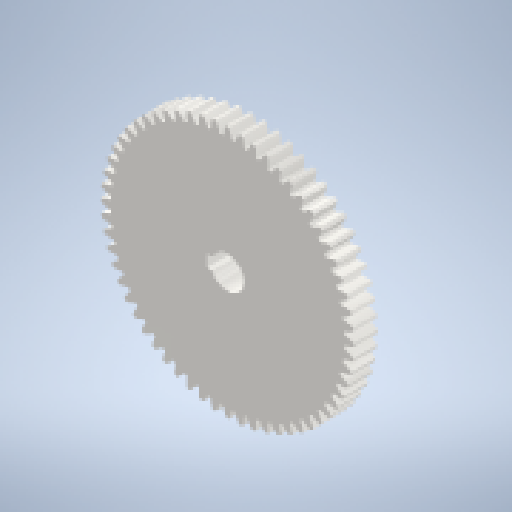
# Autodesk Inventor part: 平歯車1
Saved by Autodesk Inventor 2024 (Build 280153000, 153)
## iProperties
Created: 2023-05-30
Part Number: 平歯車1
Material: Steel
Document SubType Name: Modeling
Designer: yuta2
Categories: <?xml version="1.0" encoding="UTF-16"?> <MemberInstance><Categories><FamilyTemplate><FamilyTemplateParameter ValueType="xs:double" Id="1" ObjectReferenceKey="da_z" ObjectType="kUserParameterObject"/><FamilyTemplateParameter ValueType="xs:double" Id="2" ObjectReferenceKey="da_b" ObjectType="kUserParameterObject"/><FamilyTemplateParameter ValueType="xs:double" Id="3" ObjectReferenceKey="da_beta" ObjectType="kUserParameterObject"/><FamilyTemplateParameter ValueType="xs:double" Id="4" ObjectReferenceKey="da_da" ObjectType="kUserParameterObject"/><FamilyTemplateParameter ValueType="xs:double" Id="5" ObjectReferenceKey="da_aw" ObjectType="kUserParameterObject"/><FamilyTemplateParameter ValueType="xs:string" Id="6" ObjectReferenceKey="EAIAABAAAACIAQAAAAAAAIAAAAAAAAAA" ObjectType="83910656" SubObjectId="SurfaceGeometry"/></FamilyTemplate><ParamToTemplateMap><ParamToTemplate CategoryParameter="//CategoryParameter[@InternalName='046C89C9-8512-4d59-83FE-43B91F4F132A']" TemplateParameter="1"/><ParamToTemplate CategoryParameter="//CategoryParameter[@InternalName='2552DF32-E462-4b46-AEBF-C6C7768E72AC']" TemplateParameter="2"/><ParamToTemplate CategoryParameter="//CategoryParameter[@InternalName='C9EE641D-15FC-4fae-A226-E94C4372FDD7']" TemplateParameter="3"/><ParamToTemplate><ParamToTemplate CategoryParameter="//CategoryParameter[@InternalName='00B6519A-459B-49c7-AD84-2E56D39A5744']" ConstantValue="0.000000"/></ParamToTemplate><ParamToTemplate><ParamToTemplate CategoryParameter="//CategoryParameter[@InternalName='04B31F0E-C7A6-4894-AA32-9629BEFACF47']" ConstantValue="1.000000"/></ParamToTemplate><ParamToTemplate><ParamToTemplate CategoryParameter="//CategoryParameter[@InternalName='43CBEC2E-7847-49e7-A936-2F7889FCB2D9']" ConstantValue="0.250000"/></ParamToTemplate><ParamToTemplate><ParamToTemplate CategoryParameter="//CategoryParameter[@InternalName='B1EFC894-105D-4ebd-86BF-FA20ED196853']" ConstantValue="0.350000"/></ParamToTemplate><ParamToTemplate><ParamToTemplate CategoryParameter="//CategoryParameter[@InternalName='51175063-3D10-4879-93E8-6246FE8B403D']" ConstantValue="2060000000.000000"/></ParamToTemplate><ParamToTemplate><ParamToTemplate CategoryParameter="//CategoryParameter[@InternalName='A3A52E27-4454-46a9-B0BD-C932399B70AF']" ConstantValue="0.300000"/></ParamToTemplate><ParamToTemplate><ParamToTemplate CategoryParameter="//CategoryParameter[@InternalName='91B76062-C214-41d9-B1B9-14D2AB99603D']" ConstantValue="0.100000"/></ParamToTemplate><ParamToTemplate><ParamToTemplate CategoryParameter="//CategoryParameter[@InternalName='374E806E-8B8A-4dda-A9AA-1039D6500AD2']" ConstantValue="10.000000"/></ParamToTemplate><ParamToTemplate><ParamToTemplate CategoryParameter="//CategoryParameter[@InternalName='2D373A89-B862-43d6-8D0B-0CBF12AB9F6C']" ConstantValue="0.349066"/></ParamToTemplate><ParamToTemplate CategoryParameter="//CategoryParameter[@InternalName='37777632-D6A2-4fac-9D53-DB8ACD95C989']" TemplateParameter="4"/><ParamToTemplate CategoryParameter="//CategoryParameter[@InternalName='FD1017F1-B727-4f7e-9707-0F86F1FF9423']" TemplateParameter="5"/><ParamToTemplate><ParamToTemplate CategoryParameter="//CategoryParameter[@InternalName='9E1B4470-B2D3-4ff1-B813-535BB4CDF51A']" ConstantValue="3520000.000000"/></ParamToTemplate><ParamToTemplate><ParamToTemplate CategoryParameter="//CategoryParameter[@InternalName='F8452263-BFF6-458c-9FB1-07C4B99E95CD']" ConstantValue="11400000.000000"/></ParamToTemplate><ParamToTemplate><ParamToTemplate CategoryParameter="//CategoryParameter[@InternalName='3E3BB259-FD49-497f-8171-6EBC954A3479']" ConstantValue="2.000000"/></ParamToTemplate><ParamToTemplate CategoryParameter="//CategoryParameter[@InternalName='27C3BAF2-7550-4e4b-AE2C-0DB134B7D9B7']" TemplateParameter="6"/></ParamToTemplateMap><Category DisplayName="Gear" InternalName="DC85795E-93AB-48d5-8EEE-5A27447B64BD" Mnemonic="Gear"><CategoryParameter DisplayName="z" InternalName="046C89C9-8512-4d59-83FE-43B91F4F132A" Mnemonic="z"/><CategoryParameter DisplayName="b" InternalName="2552DF32-E462-4b46-AEBF-C6C7768E72AC" Mnemonic="b"/><CategoryParameter DisplayName="||b|" InternalName="C9EE641D-15FC-4fae-A226-E94C4372FDD7" Mnemonic="beta"/><CategoryParameter DisplayName="x" InternalName="00B6519A-459B-49c7-AD84-2E56D39A5744" Mnemonic="x"/><CategoryParameter DisplayName="a*" InternalName="04B31F0E-C7A6-4894-AA32-9629BEFACF47" Mnemonic="a"/><CategoryParameter DisplayName="c*" InternalName="43CBEC2E-7847-49e7-A936-2F7889FCB2D9" Mnemonic="c"/><CategoryParameter DisplayName="r|.f|*" InternalName="B1EFC894-105D-4ebd-86BF-FA20ED196853" Mnemonic="rf"/><CategoryParameter DisplayName="E" InternalName="51175063-3D10-4879-93E8-6246FE8B403D" Mnemonic="E"/><CategoryParameter DisplayName="||m|" InternalName="A3A52E27-4454-46a9-B0BD-C932399B70AF" Mnemonic="mi"/><Category DisplayName="SpurGear" InternalName="26C5A22E-A91E-4dfd-A3B3-23CCAFAE1764" Mnemonic="SpurGear"><CategoryParameter DisplayName="m" InternalName="91B76062-C214-41d9-B1B9-14D2AB99603D" Mnemonic="m"/><CategoryParameter DisplayName="P" InternalName="374E806E-8B8A-4dda-A9AA-1039D6500AD2" Mnemonic="PP"/><CategoryParameter DisplayName="||a|" InternalName="2D373A89-B862-43d6-8D0B-0CBF12AB9F6C" Mnemonic="alpha"/><CategoryParameter DisplayName="d|.a|" InternalName="37777632-D6A2-4fac-9D53-DB8ACD95C989" Mnemonic="da"/><CategoryParameter DisplayName="a|.w|" InternalName="FD1017F1-B727-4f7e-9707-0F86F1FF9423" Mnemonic="aw"/><CategoryParameter DisplayName="||s||.Flim|" InternalName="9E1B4470-B2D3-4ff1-B813-535BB4CDF51A" Mnemonic="sFlim"/><CategoryParameter DisplayName="||s||.Hlim|" InternalName="F8452263-BFF6-458c-9FB1-07C4B99E95CD" Mnemonic="sHlim"/><CategoryParameter DisplayName="タイプ" InternalName="3E3BB259-FD49-497f-8171-6EBC954A3479" Mnemonic="type"/><CategoryParameter DisplayName="PitchDiameter" InternalName="27C3BAF2-7550-4e4b-AE2C-0DB134B7D9B7" Mnemonic="IDS_PITCHDIAM"/></Category></Category></Categories></MemberInstance>
Density: 1 g/cm^3
Appearance: Steel
CustomPartVersion: 1
Author: yuta2
Autodesk Inventor part; units mm, degrees
sketch "Sketch1" plane through (0, 0, 0) normal (0, 0, 1) x (1, 0, 0)
  circle A0 centre (0, 0) radius 31
  dimension "d0" = 62
  constraints: 1 centre point
  measures "d0" diameter of A0
extrude "Extrusion1" add sketch "Sketch1" along normal blind 6
ref_plane "Work Plane2" through (0, 0, 3) normal (0, 0, 1) x (1, 0, 0)
sketch "Sketch2" plane through (0, 0, 0) normal (0, 0, -1) x (-1, 0, 0)
  circle A0 centre (0, 0) radius 31 projected
  circle A1 centre (0, 0) radius 30
  dimension "d3" = 60
  constraints: 1 centre point, 1 coincident
  measures "d3" diameter of A1
surface extrude "ピッチ円直径" sketch "Sketch2" against normal through all shown no curves A1
ref_plane "Work Plane8" through (0, 0, 0) normal (0.9986295, 0.052336, 0) x (0, 0, 1)
ref_plane "Work Plane9" through (0, 0, 0) normal (1, 0, 0) x (0, 1, 0)
spur gear teeth "平歯車" teeth 60 pitch diameter 60 tip diameter 62 root diameter 57.5 face width 6 start plane through (0, 0, 0) normal (0, 0, -1) x (-1, 0, 0)
sketch "スケッチ3" plane through (0, 0, 0) normal (0, 0, -1) x (-1, 0, 0)
  point P0 (0, 0)
  point P1 (0, 0)
  constraints: 1 coincident
hole "穴1" at (0, 0, 0) direction (0, 0, 1) diameter 8 end through all
sketch "スケッチ4" plane through (0, 0, 0) normal (0, 0, -1) x (-1, 0, 0)
  circle A0 centre (0, 0) radius 4 projected
  arc A1 (4.1254, 28.4525) -> (3.6437, 30.7851) centre (-8.4184, 27.0779) ccw projected
  arc A2 (3.6437, 30.7851) -> (2.8366, 30.87) centre (0, 0) ccw projected
  arc A3 (2.8366, 30.87) -> (1.8803, 28.6884) centre (13.8643, 24.7359) ccw projected
  arc A4 (1.8803, 28.6884) -> (1.1287, 28.7278) centre (0, 0) ccw projected
  arc A5 (1.1287, 28.7278) -> (0.4058, 30.9973) centre (-11.2027, 26.0496) ccw projected
  arc A6 (0.4058, 30.9973) -> (-0.4058, 30.9973) centre (0, 0) ccw projected
  arc A7 (-0.4058, 30.9973) -> (-1.1287, 28.7278) centre (11.2027, 26.0496) ccw projected
  arc A8 (-1.1287, 28.7278) -> (-1.8803, 28.6884) centre (0, 0) ccw projected
  arc A9 (-1.8803, 28.6884) -> (-2.8366, 30.87) centre (-13.8643, 24.7359) ccw projected
  arc A10 (-2.8366, 30.87) -> (-3.6437, 30.7851) centre (0, 0) ccw projected
  arc A11 (-3.6437, 30.7851) -> (-4.1254, 28.4525) centre (8.4184, 27.0779) ccw projected
  arc A12 (-4.1254, 28.4525) -> (-4.8688, 28.3347) centre (0, 0) ccw projected
  arc A13 (-4.8688, 28.3347) -> (-6.0478, 30.4043) centre (-16.3739, 23.1512) ccw projected
  arc A14 (-6.0478, 30.4043) -> (-6.8416, 30.2356) centre (0, 0) ccw projected
  arc A15 (-6.8416, 30.2356) -> (-7.0769, 27.8654) centre (5.5419, 27.8095) ccw projected
  arc A16 (-7.0769, 27.8654) -> (-7.8039, 27.6706) centre (0, 0) ccw projected
  arc A17 (-7.8039, 27.6706) -> (-9.1928, 29.6056) centre (-18.7042, 21.3128) ccw projected
  arc A18 (-9.1928, 29.6056) -> (-9.9646, 29.3548) centre (0, 0) ccw projected
  arc A19 (-9.9646, 29.3548) -> (-9.9509, 26.973) centre (2.6046, 28.2365) ccw projected
  arc A20 (-9.9509, 26.973) -> (-10.6535, 26.7033) centre (0, 0) ccw projected
  arc A21 (-10.6535, 26.7033) -> (-12.2371, 28.4825) centre (-20.8295, 19.241) ccw projected
  arc A22 (-12.2371, 28.4825) -> (-12.9785, 28.1524) centre (0, 0) ccw projected
  arc A23 (-12.9785, 28.1524) -> (-12.7158, 25.7851) centre (-0.3611, 28.3541) ccw projected
  arc A24 (-12.7158, 25.7851) -> (-13.3864, 25.4434) centre (0, 0) ccw projected
  arc A25 (-13.3864, 25.4434) -> (-15.1473, 27.0474) centre (-22.7266, 16.9583) ccw projected
  arc A26 (-15.1473, 27.0474) -> (-15.8501, 26.6416) centre (0, 0) ccw projected
  arc A27 (-15.8501, 26.6416) -> (-15.3414, 24.3147) centre (-3.323, 28.161) ccw projected
  arc A28 (-15.3414, 24.3147) -> (-15.9726, 23.9048) centre (0, 0) ccw projected
  arc A29 (-15.9726, 23.9048) -> (-17.8915, 25.3159) centre (-24.3748, 14.4898) ccw projected
  arc A30 (-17.8915, 25.3159) -> (-18.5481, 24.8389) centre (0, 0) ccw projected
  arc A31 (-18.5481, 24.8389) -> (-17.799, 22.5779) centre (-6.2484, 27.6594) ccw projected
  arc A32 (-17.799, 22.5779) -> (-18.3839, 22.1042) centre (0, 0) ccw projected
  arc A33 (-18.3839, 22.1042) -> (-20.4397, 23.307) centre (-25.7558, 11.8626) ccw projected
  arc A34 (-20.4397, 23.307) -> (-21.0428, 22.764) centre (0, 0) ccw projected
  arc A35 (-21.0428, 22.764) -> (-20.0615, 20.5937) centre (-9.1054, 26.8547) ccw projected
  arc A36 (-20.0615, 20.5937) -> (-20.5937, 20.0615) centre (0, 0) ccw projected
  arc A37 (-20.5937, 20.0615) -> (-22.764, 21.0428) centre (-26.8547, 9.1054) ccw projected
  arc A38 (-22.764, 21.0428) -> (-23.307, 20.4397) centre (0, 0) ccw projected
  arc A39 (-23.307, 20.4397) -> (-22.1042, 18.3839) centre (-11.8626, 25.7558) ccw projected
  arc A40 (-22.1042, 18.3839) -> (-22.5779, 17.799) centre (0, 0) ccw projected
  arc A41 (-22.5779, 17.799) -> (-24.8389, 18.5481) centre (-27.6594, 6.2484) ccw projected
  arc A42 (-24.8389, 18.5481) -> (-25.3159, 17.8915) centre (0, 0) ccw projected
  arc A43 (-25.3159, 17.8915) -> (-23.9048, 15.9726) centre (-14.4898, 24.3748) ccw projected
  arc A44 (-23.9048, 15.9726) -> (-24.3147, 15.3414) centre (0, 0) ccw projected
  arc A45 (-24.3147, 15.3414) -> (-26.6416, 15.8501) centre (-28.161, 3.323) ccw projected
  arc A46 (-26.6416, 15.8501) -> (-27.0474, 15.1473) centre (0, 0) ccw projected
  arc A47 (-27.0474, 15.1473) -> (-25.4434, 13.3864) centre (-16.9583, 22.7266) ccw projected
  arc A48 (-25.4434, 13.3864) -> (-25.7851, 12.7158) centre (0, 0) ccw projected
  arc A49 (-25.7851, 12.7158) -> (-28.1524, 12.9785) centre (-28.3541, 0.3611) ccw projected
  arc A50 (-28.1524, 12.9785) -> (-28.4825, 12.2371) centre (0, 0) ccw projected
  arc A51 (-28.4825, 12.2371) -> (-26.7033, 10.6535) centre (-19.241, 20.8295) ccw projected
  arc A52 (-26.7033, 10.6535) -> (-26.973, 9.9509) centre (0, 0) ccw projected
  arc A53 (-26.973, 9.9509) -> (-29.3548, 9.9646) centre (-28.2365, -2.6046) ccw projected
  arc A54 (-29.3548, 9.9646) -> (-29.6056, 9.1928) centre (0, 0) ccw projected
  arc A55 (-29.6056, 9.1928) -> (-27.6706, 7.8039) centre (-21.3128, 18.7042) ccw projected
  arc A56 (-27.6706, 7.8039) -> (-27.8654, 7.0769) centre (0, 0) ccw projected
  arc A57 (-27.8654, 7.0769) -> (-30.2356, 6.8416) centre (-27.8095, -5.5419) ccw projected
  arc A58 (-30.2356, 6.8416) -> (-30.4043, 6.0478) centre (0, 0) ccw projected
  arc A59 (-30.4043, 6.0478) -> (-28.3347, 4.8688) centre (-23.1512, 16.3739) ccw projected
  arc A60 (-28.3347, 4.8688) -> (-28.4525, 4.1254) centre (0, 0) ccw projected
  arc A61 (-28.4525, 4.1254) -> (-30.7851, 3.6437) centre (-27.0779, -8.4184) ccw projected
  arc A62 (-30.7851, 3.6437) -> (-30.87, 2.8366) centre (0, 0) ccw projected
  arc A63 (-30.87, 2.8366) -> (-28.6884, 1.8803) centre (-24.7359, 13.8643) ccw projected
  arc A64 (-28.6884, 1.8803) -> (-28.7278, 1.1287) centre (0, 0) ccw projected
  arc A65 (-28.7278, 1.1287) -> (-30.9973, 0.4058) centre (-26.0496, -11.2027) ccw projected
  arc A66 (-30.9973, 0.4058) -> (-30.9973, -0.4058) centre (0, 0) ccw projected
  arc A67 (-30.9973, -0.4058) -> (-28.7278, -1.1287) centre (-26.0496, 11.2027) ccw projected
  arc A68 (-28.7278, -1.1287) -> (-28.6884, -1.8803) centre (0, 0) ccw projected
  arc A69 (-28.6884, -1.8803) -> (-30.87, -2.8366) centre (-24.7359, -13.8643) ccw projected
  arc A70 (-30.87, -2.8366) -> (-30.7851, -3.6437) centre (0, 0) ccw projected
  arc A71 (-30.7851, -3.6437) -> (-28.4525, -4.1254) centre (-27.0779, 8.4184) ccw projected
  arc A72 (-28.4525, -4.1254) -> (-28.3347, -4.8688) centre (0, 0) ccw projected
  arc A73 (-28.3347, -4.8688) -> (-30.4043, -6.0478) centre (-23.1512, -16.3739) ccw projected
  arc A74 (-30.4043, -6.0478) -> (-30.2356, -6.8416) centre (0, 0) ccw projected
  arc A75 (-30.2356, -6.8416) -> (-27.8654, -7.0769) centre (-27.8095, 5.5419) ccw projected
  arc A76 (-27.8654, -7.0769) -> (-27.6706, -7.8039) centre (0, 0) ccw projected
  arc A77 (-27.6706, -7.8039) -> (-29.6056, -9.1928) centre (-21.3128, -18.7042) ccw projected
  arc A78 (-29.6056, -9.1928) -> (-29.3548, -9.9646) centre (0, 0) ccw projected
  arc A79 (-29.3548, -9.9646) -> (-26.973, -9.9509) centre (-28.2365, 2.6046) ccw projected
  arc A80 (-26.973, -9.9509) -> (-26.7033, -10.6535) centre (0, 0) ccw projected
  arc A81 (-26.7033, -10.6535) -> (-28.4825, -12.2371) centre (-19.241, -20.8295) ccw projected
  arc A82 (-28.4825, -12.2371) -> (-28.1524, -12.9785) centre (0, 0) ccw projected
  arc A83 (-28.1524, -12.9785) -> (-25.7851, -12.7158) centre (-28.3541, -0.3611) ccw projected
  arc A84 (-25.7851, -12.7158) -> (-25.4434, -13.3864) centre (0, 0) ccw projected
  arc A85 (-25.4434, -13.3864) -> (-27.0474, -15.1473) centre (-16.9583, -22.7266) ccw projected
  arc A86 (-27.0474, -15.1473) -> (-26.6416, -15.8501) centre (0, 0) ccw projected
  arc A87 (-26.6416, -15.8501) -> (-24.3147, -15.3414) centre (-28.161, -3.323) ccw projected
  arc A88 (-24.3147, -15.3414) -> (-23.9048, -15.9726) centre (0, 0) ccw projected
  arc A89 (-23.9048, -15.9726) -> (-25.3159, -17.8915) centre (-14.4898, -24.3748) ccw projected
  arc A90 (-25.3159, -17.8915) -> (-24.8389, -18.5481) centre (0, 0) ccw projected
  arc A91 (-24.8389, -18.5481) -> (-22.5779, -17.799) centre (-27.6594, -6.2484) ccw projected
  arc A92 (-22.5779, -17.799) -> (-22.1042, -18.3839) centre (0, 0) ccw projected
  arc A93 (-22.1042, -18.3839) -> (-23.307, -20.4397) centre (-11.8626, -25.7558) ccw projected
  arc A94 (-23.307, -20.4397) -> (-22.764, -21.0428) centre (0, 0) ccw projected
  arc A95 (-22.764, -21.0428) -> (-20.5937, -20.0615) centre (-26.8547, -9.1054) ccw projected
  arc A96 (-20.5937, -20.0615) -> (-20.0615, -20.5937) centre (0, 0) ccw projected
  arc A97 (-20.0615, -20.5937) -> (-21.0428, -22.764) centre (-9.1054, -26.8547) ccw projected
  arc A98 (-21.0428, -22.764) -> (-20.4397, -23.307) centre (0, 0) ccw projected
  arc A99 (-20.4397, -23.307) -> (-18.3839, -22.1042) centre (-25.7558, -11.8626) ccw projected
  arc A100 (-18.3839, -22.1042) -> (-17.799, -22.5779) centre (0, 0) ccw projected
  arc A101 (-17.799, -22.5779) -> (-18.5481, -24.8389) centre (-6.2484, -27.6594) ccw projected
  arc A102 (-18.5481, -24.8389) -> (-17.8915, -25.3159) centre (0, 0) ccw projected
  arc A103 (-17.8915, -25.3159) -> (-15.9726, -23.9048) centre (-24.3748, -14.4898) ccw projected
  arc A104 (-15.9726, -23.9048) -> (-15.3414, -24.3147) centre (0, 0) ccw projected
  arc A105 (-15.3414, -24.3147) -> (-15.8501, -26.6416) centre (-3.323, -28.161) ccw projected
  arc A106 (-15.8501, -26.6416) -> (-15.1473, -27.0474) centre (0, 0) ccw projected
  arc A107 (-15.1473, -27.0474) -> (-13.3864, -25.4434) centre (-22.7266, -16.9583) ccw projected
  arc A108 (-13.3864, -25.4434) -> (-12.7158, -25.7851) centre (0, 0) ccw projected
  arc A109 (-12.7158, -25.7851) -> (-12.9785, -28.1524) centre (-0.3611, -28.3541) ccw projected
  arc A110 (-12.9785, -28.1524) -> (-12.2371, -28.4825) centre (0, 0) ccw projected
  arc A111 (-12.2371, -28.4825) -> (-10.6535, -26.7033) centre (-20.8295, -19.241) ccw projected
  arc A112 (-10.6535, -26.7033) -> (-9.9509, -26.973) centre (0, 0) ccw projected
  arc A113 (-9.9509, -26.973) -> (-9.9646, -29.3548) centre (2.6046, -28.2365) ccw projected
  arc A114 (-9.9646, -29.3548) -> (-9.1928, -29.6056) centre (0, 0) ccw projected
  arc A115 (-9.1928, -29.6056) -> (-7.8039, -27.6706) centre (-18.7042, -21.3128) ccw projected
  arc A116 (-7.8039, -27.6706) -> (-7.0769, -27.8654) centre (0, 0) ccw projected
  arc A117 (-7.0769, -27.8654) -> (-6.8416, -30.2356) centre (5.5419, -27.8095) ccw projected
  arc A118 (-6.8416, -30.2356) -> (-6.0478, -30.4043) centre (0, 0) ccw projected
  arc A119 (-6.0478, -30.4043) -> (-4.8688, -28.3347) centre (-16.3739, -23.1512) ccw projected
  arc A120 (-4.8688, -28.3347) -> (-4.1254, -28.4525) centre (0, 0) ccw projected
  arc A121 (-4.1254, -28.4525) -> (-3.6437, -30.7851) centre (8.4184, -27.0779) ccw projected
  arc A122 (-3.6437, -30.7851) -> (-2.8366, -30.87) centre (0, 0) ccw projected
  arc A123 (-2.8366, -30.87) -> (-1.8803, -28.6884) centre (-13.8643, -24.7359) ccw projected
  arc A124 (-1.8803, -28.6884) -> (-1.1287, -28.7278) centre (0, 0) ccw projected
  arc A125 (-1.1287, -28.7278) -> (-0.4058, -30.9973) centre (11.2027, -26.0496) ccw projected
  arc A126 (-0.4058, -30.9973) -> (0.4058, -30.9973) centre (0, 0) ccw projected
  arc A127 (0.4058, -30.9973) -> (1.1287, -28.7278) centre (-11.2027, -26.0496) ccw projected
  arc A128 (1.1287, -28.7278) -> (1.8803, -28.6884) centre (0, 0) ccw projected
  arc A129 (1.8803, -28.6884) -> (2.8366, -30.87) centre (13.8643, -24.7359) ccw projected
  arc A130 (2.8366, -30.87) -> (3.6437, -30.7851) centre (0, 0) ccw projected
  arc A131 (3.6437, -30.7851) -> (4.1254, -28.4525) centre (-8.4184, -27.0779) ccw projected
  arc A132 (4.1254, -28.4525) -> (4.8688, -28.3347) centre (0, 0) ccw projected
  arc A133 (4.8688, -28.3347) -> (6.0478, -30.4043) centre (16.3739, -23.1512) ccw projected
  arc A134 (6.0478, -30.4043) -> (6.8416, -30.2356) centre (0, 0) ccw projected
  arc A135 (6.8416, -30.2356) -> (7.0769, -27.8654) centre (-5.5419, -27.8095) ccw projected
  arc A136 (7.0769, -27.8654) -> (7.8039, -27.6706) centre (0, 0) ccw projected
  arc A137 (7.8039, -27.6706) -> (9.1928, -29.6056) centre (18.7042, -21.3128) ccw projected
  arc A138 (9.1928, -29.6056) -> (9.9646, -29.3548) centre (0, 0) ccw projected
  arc A139 (9.9646, -29.3548) -> (9.9509, -26.973) centre (-2.6046, -28.2365) ccw projected
  arc A140 (9.9509, -26.973) -> (10.6535, -26.7033) centre (0, 0) ccw projected
  arc A141 (10.6535, -26.7033) -> (12.2371, -28.4825) centre (20.8295, -19.241) ccw projected
  arc A142 (12.2371, -28.4825) -> (12.9785, -28.1524) centre (0, 0) ccw projected
  arc A143 (12.9785, -28.1524) -> (12.7158, -25.7851) centre (0.3611, -28.3541) ccw projected
  arc A144 (12.7158, -25.7851) -> (13.3864, -25.4434) centre (0, 0) ccw projected
  arc A145 (13.3864, -25.4434) -> (15.1473, -27.0474) centre (22.7266, -16.9583) ccw projected
  arc A146 (15.1473, -27.0474) -> (15.8501, -26.6416) centre (0, 0) ccw projected
  arc A147 (15.8501, -26.6416) -> (15.3414, -24.3147) centre (3.323, -28.161) ccw projected
  arc A148 (15.3414, -24.3147) -> (15.9726, -23.9048) centre (0, 0) ccw projected
  arc A149 (15.9726, -23.9048) -> (17.8915, -25.3159) centre (24.3748, -14.4898) ccw projected
  arc A150 (17.8915, -25.3159) -> (18.5481, -24.8389) centre (0, 0) ccw projected
  arc A151 (18.5481, -24.8389) -> (17.799, -22.5779) centre (6.2484, -27.6594) ccw projected
  arc A152 (17.799, -22.5779) -> (18.3839, -22.1042) centre (0, 0) ccw projected
  arc A153 (18.3839, -22.1042) -> (20.4397, -23.307) centre (25.7558, -11.8626) ccw projected
  arc A154 (20.4397, -23.307) -> (21.0428, -22.764) centre (0, 0) ccw projected
  arc A155 (21.0428, -22.764) -> (20.0615, -20.5937) centre (9.1054, -26.8547) ccw projected
  arc A156 (20.0615, -20.5937) -> (20.5937, -20.0615) centre (0, 0) ccw projected
  arc A157 (20.5937, -20.0615) -> (22.764, -21.0428) centre (26.8547, -9.1054) ccw projected
  arc A158 (22.764, -21.0428) -> (23.307, -20.4397) centre (0, 0) ccw projected
  arc A159 (23.307, -20.4397) -> (22.1042, -18.3839) centre (11.8626, -25.7558) ccw projected
  arc A160 (22.1042, -18.3839) -> (22.5779, -17.799) centre (0, 0) ccw projected
  arc A161 (22.5779, -17.799) -> (24.8389, -18.5481) centre (27.6594, -6.2484) ccw projected
  arc A162 (24.8389, -18.5481) -> (25.3159, -17.8915) centre (0, 0) ccw projected
  arc A163 (25.3159, -17.8915) -> (23.9048, -15.9726) centre (14.4898, -24.3748) ccw projected
  arc A164 (23.9048, -15.9726) -> (24.3147, -15.3414) centre (0, 0) ccw projected
  arc A165 (24.3147, -15.3414) -> (26.6416, -15.8501) centre (28.161, -3.323) ccw projected
  arc A166 (26.6416, -15.8501) -> (27.0474, -15.1473) centre (0, 0) ccw projected
  arc A167 (27.0474, -15.1473) -> (25.4434, -13.3864) centre (16.9583, -22.7266) ccw projected
  arc A168 (25.4434, -13.3864) -> (25.7851, -12.7158) centre (0, 0) ccw projected
  arc A169 (25.7851, -12.7158) -> (28.1524, -12.9785) centre (28.3541, -0.3611) ccw projected
  arc A170 (28.1524, -12.9785) -> (28.4825, -12.2371) centre (0, 0) ccw projected
  arc A171 (28.4825, -12.2371) -> (26.7033, -10.6535) centre (19.241, -20.8295) ccw projected
  arc A172 (26.7033, -10.6535) -> (26.973, -9.9509) centre (0, 0) ccw projected
  arc A173 (26.973, -9.9509) -> (29.3548, -9.9646) centre (28.2365, 2.6046) ccw projected
  arc A174 (29.3548, -9.9646) -> (29.6056, -9.1928) centre (0, 0) ccw projected
  arc A175 (29.6056, -9.1928) -> (27.6706, -7.8039) centre (21.3128, -18.7042) ccw projected
  arc A176 (27.6706, -7.8039) -> (27.8654, -7.0769) centre (0, 0) ccw projected
  arc A177 (27.8654, -7.0769) -> (30.2356, -6.8416) centre (27.8095, 5.5419) ccw projected
  arc A178 (30.2356, -6.8416) -> (30.4043, -6.0478) centre (0, 0) ccw projected
  arc A179 (30.4043, -6.0478) -> (28.3347, -4.8688) centre (23.1512, -16.3739) ccw projected
  arc A180 (28.3347, -4.8688) -> (28.4525, -4.1254) centre (0, 0) ccw projected
  arc A181 (28.4525, -4.1254) -> (30.7851, -3.6437) centre (27.0779, 8.4184) ccw projected
  arc A182 (30.7851, -3.6437) -> (30.87, -2.8366) centre (0, 0) ccw projected
  arc A183 (30.87, -2.8366) -> (28.6884, -1.8803) centre (24.7359, -13.8643) ccw projected
  arc A184 (28.6884, -1.8803) -> (28.7278, -1.1287) centre (0, 0) ccw projected
  arc A185 (28.7278, -1.1287) -> (30.9973, -0.4058) centre (26.0496, 11.2027) ccw projected
  arc A186 (30.9973, -0.4058) -> (30.9973, 0.4058) centre (0, 0) ccw projected
  arc A187 (30.9973, 0.4058) -> (28.7278, 1.1287) centre (26.0496, -11.2027) ccw projected
  arc A188 (28.7278, 1.1287) -> (28.6884, 1.8803) centre (0, 0) ccw projected
  arc A189 (28.6884, 1.8803) -> (30.87, 2.8366) centre (24.7359, 13.8643) ccw projected
  arc A190 (30.87, 2.8366) -> (30.7851, 3.6437) centre (0, 0) ccw projected
  arc A191 (30.7851, 3.6437) -> (28.4525, 4.1254) centre (27.0779, -8.4184) ccw projected
  arc A192 (28.4525, 4.1254) -> (28.3347, 4.8688) centre (0, 0) ccw projected
  arc A193 (28.3347, 4.8688) -> (30.4043, 6.0478) centre (23.1512, 16.3739) ccw projected
  arc A194 (30.4043, 6.0478) -> (30.2356, 6.8416) centre (0, 0) ccw projected
  arc A195 (30.2356, 6.8416) -> (27.8654, 7.0769) centre (27.8095, -5.5419) ccw projected
  arc A196 (27.8654, 7.0769) -> (27.6706, 7.8039) centre (0, 0) ccw projected
  arc A197 (27.6706, 7.8039) -> (29.6056, 9.1928) centre (21.3128, 18.7042) ccw projected
  arc A198 (29.6056, 9.1928) -> (29.3548, 9.9646) centre (0, 0) ccw projected
  arc A199 (29.3548, 9.9646) -> (26.973, 9.9509) centre (28.2365, -2.6046) ccw projected
  arc A200 (26.973, 9.9509) -> (26.7033, 10.6535) centre (0, 0) ccw projected
  arc A201 (26.7033, 10.6535) -> (28.4825, 12.2371) centre (19.241, 20.8295) ccw projected
  arc A202 (28.4825, 12.2371) -> (28.1524, 12.9785) centre (0, 0) ccw projected
  arc A203 (28.1524, 12.9785) -> (25.7851, 12.7158) centre (28.3541, 0.3611) ccw projected
  arc A204 (25.7851, 12.7158) -> (25.4434, 13.3864) centre (0, 0) ccw projected
  arc A205 (25.4434, 13.3864) -> (27.0474, 15.1473) centre (16.9583, 22.7266) ccw projected
  arc A206 (27.0474, 15.1473) -> (26.6416, 15.8501) centre (0, 0) ccw projected
  arc A207 (26.6416, 15.8501) -> (24.3147, 15.3414) centre (28.161, 3.323) ccw projected
  arc A208 (24.3147, 15.3414) -> (23.9048, 15.9726) centre (0, 0) ccw projected
  arc A209 (23.9048, 15.9726) -> (25.3159, 17.8915) centre (14.4898, 24.3748) ccw projected
  arc A210 (25.3159, 17.8915) -> (24.8389, 18.5481) centre (0, 0) ccw projected
  arc A211 (24.8389, 18.5481) -> (22.5779, 17.799) centre (27.6594, 6.2484) ccw projected
  arc A212 (22.5779, 17.799) -> (22.1042, 18.3839) centre (0, 0) ccw projected
  arc A213 (22.1042, 18.3839) -> (23.307, 20.4397) centre (11.8626, 25.7558) ccw projected
  arc A214 (23.307, 20.4397) -> (22.764, 21.0428) centre (0, 0) ccw projected
  arc A215 (22.764, 21.0428) -> (20.5937, 20.0615) centre (26.8547, 9.1054) ccw projected
  arc A216 (20.5937, 20.0615) -> (20.0615, 20.5937) centre (0, 0) ccw projected
  arc A217 (20.0615, 20.5937) -> (21.0428, 22.764) centre (9.1054, 26.8547) ccw projected
  arc A218 (21.0428, 22.764) -> (20.4397, 23.307) centre (0, 0) ccw projected
  arc A219 (20.4397, 23.307) -> (18.3839, 22.1042) centre (25.7558, 11.8626) ccw projected
  arc A220 (18.3839, 22.1042) -> (17.799, 22.5779) centre (0, 0) ccw projected
  arc A221 (17.799, 22.5779) -> (18.5481, 24.8389) centre (6.2484, 27.6594) ccw projected
  arc A222 (18.5481, 24.8389) -> (17.8915, 25.3159) centre (0, 0) ccw projected
  arc A223 (17.8915, 25.3159) -> (15.9726, 23.9048) centre (24.3748, 14.4898) ccw projected
  arc A224 (15.9726, 23.9048) -> (15.3414, 24.3147) centre (0, 0) ccw projected
  arc A225 (15.3414, 24.3147) -> (15.8501, 26.6416) centre (3.323, 28.161) ccw projected
  arc A226 (15.8501, 26.6416) -> (15.1473, 27.0474) centre (0, 0) ccw projected
  arc A227 (15.1473, 27.0474) -> (13.3864, 25.4434) centre (22.7266, 16.9583) ccw projected
  arc A228 (13.3864, 25.4434) -> (12.7158, 25.7851) centre (0, 0) ccw projected
  arc A229 (12.7158, 25.7851) -> (12.9785, 28.1524) centre (0.3611, 28.3541) ccw projected
  arc A230 (12.9785, 28.1524) -> (12.2371, 28.4825) centre (0, 0) ccw projected
  arc A231 (12.2371, 28.4825) -> (10.6535, 26.7033) centre (20.8295, 19.241) ccw projected
  arc A232 (10.6535, 26.7033) -> (9.9509, 26.973) centre (0, 0) ccw projected
  arc A233 (9.9509, 26.973) -> (9.9646, 29.3548) centre (-2.6046, 28.2365) ccw projected
  arc A234 (9.9646, 29.3548) -> (9.1928, 29.6056) centre (0, 0) ccw projected
  arc A235 (9.1928, 29.6056) -> (7.8039, 27.6706) centre (18.7042, 21.3128) ccw projected
  arc A236 (7.8039, 27.6706) -> (7.0769, 27.8654) centre (0, 0) ccw projected
  arc A237 (7.0769, 27.8654) -> (6.8416, 30.2356) centre (-5.5419, 27.8095) ccw projected
  arc A238 (6.8416, 30.2356) -> (6.0478, 30.4043) centre (0, 0) ccw projected
  arc A239 (6.0478, 30.4043) -> (4.8688, 28.3347) centre (16.3739, 23.1512) ccw projected
  arc A240 (4.8688, 28.3347) -> (4.1254, 28.4525) centre (0, 0) ccw projected
  circle A241 centre (0, 0) radius 17.5
  dimension "d56" = 35
  constraints: 1 centre point, 1 coincident
  measures "d56" diameter of A241
extrude "押し出し2" add sketch "スケッチ4" along normal blind 8 contours A241
sketch "スケッチ5" plane through (0, 0, -8) normal (0, 0, -1) x (-1, 0, 0)
  circle A0 centre (0, 0) radius 4 projected
  line L0 (3.7081, 1.5) -> (5.1081, 1.5)
  line L1 (5.1081, 1.5) -> (5.1081, -1.5)
  line L2 (5.1081, -1.5) -> (3.7081, -1.5)
  line L3 (3.7081, -1.5) -> (3.7081, 1.5)
  circle A1 centre (0, 0) radius 4 projected
  dimension "d59" = 3
  dimension "d60" = 1.4
  constraints: 8 end point, 2 parallel, 1 horizontal, 1 perpendicular, 1 point on circle, 2 other
  measures "d59" distance of L0.end L1.end
  measures "d60" distance of L1.end L2.end
extrude "押し出し3" cut sketch "スケッチ5" against normal through all contours A0 L0 L1 L2
equation "\"d0\" = da_da"
equation "\"d1\" = da_b"
equation "\"d3\" = da_d"
equation "\"d16\" = da_aw"
equation "\"d43\" = da_aw"
equation "\"d46\" = da_aw"
equation "\"da_da\" = 62"
equation "\"da_b\" = 6"
equation "\"da_d\" = 60"
equation "\"da_aw\" = 58.5"
body "Solid1"
body "Srf1"
